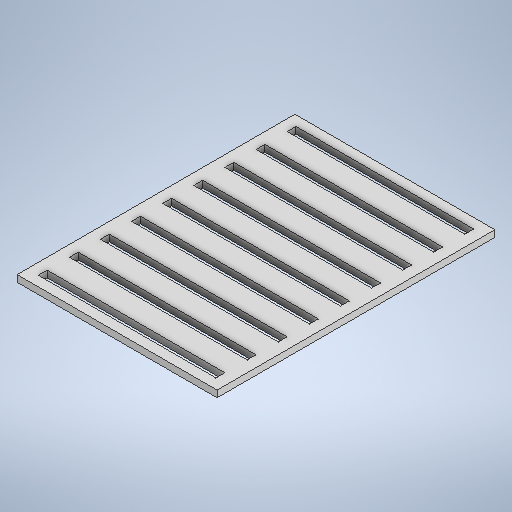
# Autodesk Inventor part: flood tray_2
Saved by Autodesk Inventor 2025 (Build 290162000, 162)
## iProperties
Created: 2024-07-12
Part Number: flood tray_2
Material: Generic
Document SubType Name: Modeling
Designer: User
Density: 1 g/cm^3
Appearance: Default
Author: User
Autodesk Inventor part; units mm, degrees
ref_plane "YZ Plane" through (0, 0, 0) normal (1, 0, 0) x (0, 1, 0)
ref_plane "XZ Plane" through (0, 0, 0) normal (0, 1, 0) x (-1, 0, 0)
ref_plane "XY Plane" through (0, 0, 0) normal (0, 0, 1) x (1, 0, 0)
sketch "Sketch1" plane through (0, 0, 0) normal (0, 1, 0) x (-1, 0, 0)
  line L0 (-450, 625) -> (450, 625)
  line L1 (450, 625) -> (450, -625)
  line L2 (450, -625) -> (-450, -625)
  line L3 (-450, -625) -> (-450, 625)
  line L4 (-450, 625) -> (450, -625) construction
  line L5 (450, 625) -> (-450, -625) construction
  line L6 (400, 580) -> (-400, 580)
  line L7 (-400, 580) -> (-400, 540)
  line L8 (-400, 540) -> (400, 540)
  line L9 (400, 540) -> (400, 580)
  line L10 (400, 580) -> (-400, 540) construction
  line L11 (-400, 580) -> (400, 540) construction
  line L12 (400, 440) -> (-400, 440)
  line L13 (-400, 440) -> (-400, 400)
  line L14 (-400, 400) -> (400, 400)
  line L15 (400, 400) -> (400, 440)
  line L16 (400, 440) -> (-400, 400) construction
  line L17 (-400, 440) -> (400, 400) construction
  line L18 (400, 300) -> (-400, 300)
  line L19 (-400, 300) -> (-400, 260)
  line L20 (-400, 260) -> (400, 260)
  line L21 (400, 260) -> (400, 300)
  line L22 (400, 300) -> (-400, 260) construction
  line L23 (-400, 300) -> (400, 260) construction
  line L24 (400, 160) -> (-400, 160)
  line L25 (-400, 160) -> (-400, 120)
  line L26 (-400, 120) -> (400, 120)
  line L27 (400, 120) -> (400, 160)
  line L28 (400, 160) -> (-400, 120) construction
  line L29 (-400, 160) -> (400, 120) construction
  line L30 (400, 20) -> (-400, 20)
  line L31 (-400, 20) -> (-400, -20)
  line L32 (-400, -20) -> (400, -20)
  line L33 (400, -20) -> (400, 20)
  line L34 (400, 20) -> (-400, -20) construction
  line L35 (-400, 20) -> (400, -20) construction
  line L36 (400, -120) -> (-400, -120)
  line L37 (-400, -120) -> (-400, -160)
  line L38 (-400, -160) -> (400, -160)
  line L39 (400, -160) -> (400, -120)
  line L40 (400, -120) -> (-400, -160) construction
  line L41 (-400, -120) -> (400, -160) construction
  line L42 (400, -260) -> (-400, -260)
  line L43 (-400, -260) -> (-400, -300)
  line L44 (-400, -300) -> (400, -300)
  line L45 (400, -300) -> (400, -260)
  line L46 (400, -260) -> (-400, -300) construction
  line L47 (-400, -260) -> (400, -300) construction
  line L48 (400, -400) -> (-400, -400)
  line L49 (-400, -400) -> (-400, -440)
  line L50 (-400, -440) -> (400, -440)
  line L51 (400, -440) -> (400, -400)
  line L52 (400, -400) -> (-400, -440) construction
  line L53 (-400, -400) -> (400, -440) construction
  line L54 (400, -540) -> (-400, -540)
  line L55 (-400, -540) -> (-400, -580)
  line L56 (-400, -580) -> (400, -580)
  line L57 (400, -580) -> (400, -540)
  line L58 (400, -540) -> (-400, -580) construction
  line L59 (-400, -540) -> (400, -580) construction
  point P0 (0, 0)
  point P1 (0, 560)
  point P2 (0, 420)
  point P3 (0, 280)
  point P4 (0, 140)
  point P5 (0, 0)
  point P6 (0, -140)
  point P7 (0, -280)
  point P8 (0, -420)
  point P9 (0, -560)
  point P10 (0, -260)
  point P11 (0, -120)
  point P12 (50, 0)
  dimension "d0" = 1250
  dimension "d1" = 900
  dimension "d2" = 800
  dimension "d3" = 40
  dimension "d7" = 40
  dimension "d9" = 40
  dimension "d10" = 45
  dimension "d11" = 100
  dimension "d12" = 100
  dimension "d14" = 40
  dimension "d16" = 40
  dimension "d18" = 40
  dimension "d20" = 40
  dimension "d22" = 40
  dimension "d24" = 40
  dimension "d27" = 100
  dimension "d28" = 100
  dimension "d29" = 100
  dimension "d30" = 100
  dimension "d31" = 100
  dimension "d32" = 100
  dimension "d36" = 50
  constraints: 120 end point, 28 parallel, 22 midpoint, 10 horizontal, 10 perpendicular, 10 vertical alignment, 1 coincident, 1 horizontal alignment
  measures "d0" distance of L0.end L1.end
  measures "d1" distance of L1.end L2.end
  measures "d2" distance of L6.start L6.end
  measures "d3" distance of L8.end L6.start
  measures "d7" distance of L14.end L12.start
  measures "d9" distance of L20.end L18.start
  measures "d10" distance between parallel lines of L0 L6
  measures "d11" distance between parallel lines of L12 L8
  measures "d12" distance between parallel lines of L18 L14
  measures "d14" distance of L26.end L24.start
  measures "d16" distance of L32.end L30.start
  measures "d18" distance of L38.end L36.start
  measures "d20" distance of L44.end L42.start
  measures "d22" distance of L50.end L48.start
  measures "d24" distance of L56.end L54.start
  measures "d27" distance between parallel lines of L20 L24
  measures "d28" distance between parallel lines of L26 L30
  measures "d29" distance between parallel lines of L32 L36
  measures "d30" distance between parallel lines of L38 L42
  measures "d31" distance between parallel lines of L44 L48
  measures "d32" distance between parallel lines of L50 L54
  measures "d36" distance of point (0, 0) point (50, 0)
extrude "Extrusion1" add sketch "Sketch1" along normal blind 30
body "Solid1"
